Autodesk Inventor part; units mm, degrees
(part 2 of 2)
ref_plane "to_L_Winkel_1_YZ" through (-98.75, 0, -61.025) normal (0, 0, -1) x (0, -1, 0)
ref_plane "to_L_Winkel_1_ZX" through (-98.75, 0, -61.025) normal (0, -1, 0) x (-1, 0, 0)
ref_plane "to_MP_XY" through (0, 0, -61.125) normal (0, 0, -1) x (1, 0, 0)
ref_plane "to_MP_YZ" through (0, 0, -61.125) normal (1, 0, 0) x (0, -1, 0)
ref_plane "to_MP_ZX" through (0, 0, -61.125) normal (0, -1, 0) x (0, 0, -1)
sketch "Esboço47" plane through (-100, 0, 0) normal (-1, 0, 0) x (0, 0, 1)
  line L0 (-30.51, -30.51) -> (30.51, -30.51)
  line L1 (30.51, -30.51) -> (30.51, 30.51)
  line L2 (30.51, 30.51) -> (-30.51, 30.51)
  line L3 (-30.51, 30.51) -> (-30.51, -30.51)
  line L4 (-30.51, -30.51) -> (30.51, 30.51) construction
  line L5 (30.51, -30.51) -> (-30.51, 30.51) construction
  point P0 (0, 0)
  dimension "d98" = 61.02
  constraints: 12 end point, 2 midpoint, 2 parallel, 2 perpendicular, 1 horizontal
  measures "d98" distance of L1.end L2.end
extrude "Extrusão22" cut sketch "Esboço47" against normal blind 10
body "Solid1"
